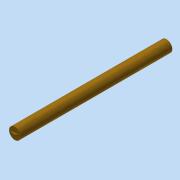
# Autodesk Inventor part: 2mmToSeal
Saved by Autodesk Inventor 2017 (Build 210142000, 142)
## iProperties
Created: 2016-12-11
Part Number: 2mmToSeal
Material: Brass, Soft Yellow, Welded
Document SubType Name: Modeling
Designer: techn
Density: 8.5 g/cm^3
Appearance: Weld - Brass
Author: techn
Autodesk Inventor part; units mm, degrees
ref_plane "YZ Plane" through (0, 0, 0) normal (1, 0, 0) x (0, 1, 0)
ref_plane "XZ Plane" through (0, 0, 0) normal (0, 1, 0) x (-1, 0, 0)
ref_plane "XY Plane" through (0, 0, 0) normal (0, 0, 1) x (1, 0, 0)
sketch "Sketch1" plane through (0, 0, 0) normal (0, 0, 1) x (1, 0, 0)
  circle A0 centre (0, 0) radius 1
  dimension "d0" = 2
  constraints: 1 centre point, 1 coincident
  measures "d0" diameter of A0
extrude "Extrusion1" add sketch "Sketch1" along normal blind 25.4
sketch "Sketch2" plane through (0, 0, 0) normal (0, 1, 0) x (-1, 0, 0)
  line L0 (1, 25.4) -> (-1, 25.4) projected
  arc A0 (1, 25.4) -> (-1, 25.4) centre (0, 25.4) ccw
  line L1 (-1, 0) -> (-1, 25.4) projected
  point P0 (0, 0)
  constraints: 2 point on circle, 1 centre point, 1 tangent
extrude "Extrusion2" add sketch "Sketch2" along normal mid plane 0.254
sketch "Sketch3" plane through (0, 0, 25.4) normal (0, 0, 1) x (1, 0, 0)
  arc A0 (0.9919, 0.127) -> (-0.9919, 0.127) centre (0, 0) ccw projected
  arc A1 (-0.9919, -0.127) -> (0.9919, -0.127) centre (0, 0) ccw projected
  circle A2 centre (0, 0) radius 1
  constraints: 1 centre point, 1 coincident, 1 concentric
extrude "Extrusion3" add sketch "Sketch3" along normal blind 0.762
body "Solid1"
